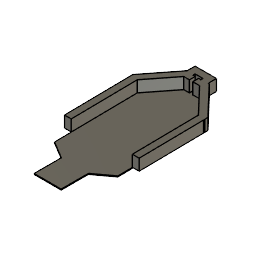
PCB CASE F3D (Autodesk Fusion 360 design; units mm, degrees)
part number: 2026-09-06-12-23-15-021
Autodesk Fusion 360 part; units mm, degrees
sketch "KiCad Dongle pcb-Edge_Cuts" plane through (0, 0, 0) normal (0, 0, 1) x (1, 0, 0)
  line L0 (141.0096, -48.4769) -> (141.0231, -48.4904)
  line L1 (141.0231, -48.4904) -> (141.025, -48.5)
  line L2 (141.025, -48.5) -> (141.025, -49.5)
  line L3 (141.025, -49.5) -> (141.0231, -49.5096)
  line L4 (141.0231, -49.5096) -> (141.0096, -49.5231)
  line L5 (141.0096, -49.5231) -> (141, -49.525)
  line L6 (141, -49.525) -> (140.025, -49.525)
  line L7 (140.025, -49.525) -> (140.025, -51.975)
  line L8 (140.025, -51.975) -> (143, -51.975)
  line L9 (143, -51.975) -> (143.0096, -51.9769)
  line L10 (143.0096, -51.9769) -> (143.0098, -51.9771)
  line L11 (143.0098, -51.9771) -> (143.0101, -51.9771)
  line L12 (143.0101, -51.9771) -> (143.0181, -51.9827)
  line L13 (143.0181, -51.9827) -> (154.0181, -63.4827)
  line L14 (154.0181, -63.4827) -> (154.0228, -63.4901)
  line L15 (154.0228, -63.4901) -> (154.0231, -63.4904)
  line L16 (154.0231, -63.4904) -> (154.0232, -63.4907)
  line L17 (154.0232, -63.4907) -> (154.0233, -63.4909)
  line L18 (154.0233, -63.4909) -> (154.0233, -63.4914)
  line L19 (154.0233, -63.4914) -> (154.025, -63.5)
  line L20 (154.025, -63.5) -> (154.025, -63.9998)
  line L21 (154.025, -63.9998) -> (154.4913, -99.4997)
  line L22 (154.4913, -99.4997) -> (154.4895, -99.5093)
  line L23 (154.4895, -99.5093) -> (154.488, -99.5108)
  line L24 (154.488, -99.5108) -> (154.4877, -99.5129)
  line L25 (154.4877, -99.5129) -> (154.4811, -99.5201)
  line L26 (154.4811, -99.5201) -> (147.025, -105.0126)
  line L27 (147.025, -105.0126) -> (147.025, -117)
  line L28 (147.025, -117) -> (147.0231, -117.0096)
  line L29 (147.0231, -117.0096) -> (147.0096, -117.0231)
  line L30 (147.0096, -117.0231) -> (147, -117.025)
  line L31 (147, -117.025) -> (135, -117.025)
  line L32 (135, -117.025) -> (134.9904, -117.0231)
  line L33 (134.9904, -117.0231) -> (134.9769, -117.0096)
  line L34 (134.9769, -117.0096) -> (134.975, -117)
  line L35 (134.975, -117) -> (134.975, -105.0142)
  line L36 (134.975, -105.0142) -> (127.4871, -100.5214)
  line L37 (127.4871, -100.5214) -> (127.4799, -100.5149)
  line L38 (127.4799, -100.5149) -> (127.4792, -100.512)
  line L39 (127.4792, -100.512) -> (127.477, -100.5099)
  line L40 (127.477, -100.5099) -> (127.475, -100.5003)
  line L41 (127.475, -100.5003) -> (126.975, -63.5003)
  line L42 (126.975, -63.5003) -> (126.9761, -63.4946)
  line L43 (126.9761, -63.4946) -> (126.9759, -63.4933)
  line L44 (126.9759, -63.4933) -> (126.9765, -63.4921)
  line L45 (126.9765, -63.4921) -> (126.9768, -63.4907)
  line L46 (126.9768, -63.4907) -> (126.9777, -63.4898)
  line L47 (126.9777, -63.4898) -> (126.9803, -63.4846)
  line L48 (126.9803, -63.4846) -> (135.9803, -51.9846)
  line L49 (135.9803, -51.9846) -> (135.9877, -51.9782)
  line L50 (135.9877, -51.9782) -> (135.9893, -51.978)
  line L51 (135.9893, -51.978) -> (135.9904, -51.9769)
  line L52 (135.9904, -51.9769) -> (136, -51.975)
  line L53 (136, -51.975) -> (138.475, -51.975)
  line L54 (138.475, -51.975) -> (138.475, -51.5)
  line L55 (138.475, -51.5) -> (138.475, -49.525)
  line L56 (138.475, -49.525) -> (137.5, -49.525)
  line L57 (137.5, -49.525) -> (137.4904, -49.5231)
  line L58 (137.4904, -49.5231) -> (137.4769, -49.5096)
  line L59 (137.4769, -49.5096) -> (137.475, -49.5)
  line L60 (137.475, -49.5) -> (137.475, -48.5)
  line L61 (137.475, -48.5) -> (137.4769, -48.4904)
  line L62 (137.4769, -48.4904) -> (137.4904, -48.4769)
  line L63 (137.4904, -48.4769) -> (137.5, -48.475)
  line L64 (137.5, -48.475) -> (141, -48.475)
  line L65 (141, -48.475) -> (141.0096, -48.4769)
  line L66 (137.525, -48.525) -> (137.525, -49.475)
  line L67 (137.525, -49.475) -> (138.5, -49.475)
  line L68 (138.5, -49.475) -> (138.5096, -49.4769)
  line L69 (138.5096, -49.4769) -> (138.5231, -49.4904)
  line L70 (138.5231, -49.4904) -> (138.525, -49.5)
  line L71 (138.525, -49.5) -> (138.525, -51.5)
  line L72 (138.525, -51.5) -> (138.525, -52)
  line L73 (138.525, -52) -> (138.5231, -52.0096)
  line L74 (138.5231, -52.0096) -> (138.5096, -52.0231)
  line L75 (138.5096, -52.0231) -> (138.5, -52.025)
  line L76 (138.5, -52.025) -> (136.0122, -52.025)
  line L77 (136.0122, -52.025) -> (127.0251, -63.5085)
  line L78 (127.0251, -63.5085) -> (127.5248, -100.4857)
  line L79 (127.5248, -100.4857) -> (135.0129, -104.9786)
  line L80 (135.0129, -104.9786) -> (135.0201, -104.9851)
  line L81 (135.0201, -104.9851) -> (135.0209, -104.9882)
  line L82 (135.0209, -104.9882) -> (135.0231, -104.9904)
  line L83 (135.0231, -104.9904) -> (135.025, -105)
  line L84 (135.025, -105) -> (135.025, -116.975)
  line L85 (135.025, -116.975) -> (146.975, -116.975)
  line L86 (146.975, -116.975) -> (146.975, -105)
  line L87 (146.975, -105) -> (146.9769, -104.9904)
  line L88 (146.9769, -104.9904) -> (146.9783, -104.989)
  line L89 (146.9783, -104.989) -> (146.9786, -104.9871)
  line L90 (146.9786, -104.9871) -> (146.9852, -104.9799)
  line L91 (146.9852, -104.9799) -> (154.4411, -99.4875)
  line L92 (154.4411, -99.4875) -> (153.975, -64.0003)
  line L93 (153.975, -64.0003) -> (153.975, -64.0002)
  line L94 (153.975, -64.0002) -> (153.975, -64)
  line L95 (153.975, -64) -> (153.975, -63.51)
  line L96 (153.975, -63.51) -> (142.9893, -52.025)
  line L97 (142.9893, -52.025) -> (140, -52.025)
  line L98 (140, -52.025) -> (139.9904, -52.0231)
  line L99 (139.9904, -52.0231) -> (139.9769, -52.0096)
  line L100 (139.9769, -52.0096) -> (139.975, -52)
  line L101 (139.975, -52) -> (139.975, -49.5)
  line L102 (139.975, -49.5) -> (139.9769, -49.4904)
  line L103 (139.9769, -49.4904) -> (139.9904, -49.4769)
  line L104 (139.9904, -49.4769) -> (140, -49.475)
  line L105 (140, -49.475) -> (140.975, -49.475)
  line L106 (140.975, -49.475) -> (140.975, -48.525)
  line L107 (140.975, -48.525) -> (137.525, -48.525)
extrude "Extrude1" add sketch "KiCad Dongle pcb-Edge_Cuts" along normal blind 0.4 contours L66 L67 L68 L69 L70 L71 L72 L73 L74 L75 L76 L77 L78 L79 L80 L81 L82 L83 L84 L85 L86 L87 L89 L90 L91 L92 L95 L96 L97 L98 L99 L100 L101 L102 L103 L104 L105 L106 L107 makes body 1
sketch "Sketch3" plane through (0, 0, 0.4) normal (0, 0, 1) x (-1, 0, 0)
  line L0 (-140.975, 48.525) -> (-137.525, 48.525)
  line L1 (-137.525, 48.525) -> (-137.525, 49.475)
  line L2 (-137.525, 49.475) -> (-138.5, 49.475)
  line L3 (-138.5, 49.475) -> (-138.5096, 49.4769)
  line L4 (-138.5096, 49.4769) -> (-138.5231, 49.4904)
  line L5 (-138.5231, 49.4904) -> (-138.525, 49.5)
  line L6 (-138.525, 49.5) -> (-138.525, 52)
  line L7 (-138.525, 52) -> (-138.5231, 52.0096)
  line L8 (-138.5231, 52.0096) -> (-138.5096, 52.0231)
  line L9 (-138.5096, 52.0231) -> (-138.5, 52.025)
  line L10 (-138.5, 52.025) -> (-136.0122, 52.025)
  line L11 (-136.0122, 52.025) -> (-127.0251, 63.5085)
  line L12 (-127.0251, 63.5085) -> (-127.5248, 100.4857)
  line L13 (-127.5248, 100.4857) -> (-135.0129, 104.9786)
  line L14 (-135.0129, 104.9786) -> (-135.0201, 104.9851)
  line L15 (-135.0201, 104.9851) -> (-135.0209, 104.9882)
  line L16 (-135.0209, 104.9882) -> (-135.0231, 104.9904)
  line L17 (-135.0231, 104.9904) -> (-135.025, 105)
  line L18 (-135.025, 105) -> (-135.025, 116.975)
  line L19 (-135.025, 116.975) -> (-146.975, 116.975)
  line L20 (-146.975, 116.975) -> (-146.975, 105)
  line L21 (-146.975, 105) -> (-146.9769, 104.9904)
  line L22 (-146.9769, 104.9904) -> (-146.9783, 104.989)
  line L23 (-146.9783, 104.989) -> (-146.9786, 104.9871)
  line L24 (-146.9786, 104.9871) -> (-146.9852, 104.9799)
  line L25 (-146.9852, 104.9799) -> (-154.4411, 99.4875)
  line L26 (-154.4411, 99.4875) -> (-153.975, 64.0003)
  line L27 (-153.975, 64.0003) -> (-153.975, 64.0002)
  line L28 (-153.975, 64.0002) -> (-153.975, 64)
  line L29 (-153.975, 64) -> (-153.975, 63.51)
  line L30 (-153.975, 63.51) -> (-142.9893, 52.025)
  line L31 (-142.9893, 52.025) -> (-140, 52.025)
  line L32 (-140, 52.025) -> (-139.9904, 52.0231)
  line L33 (-139.9904, 52.0231) -> (-139.9769, 52.0096)
  line L34 (-139.9769, 52.0096) -> (-139.975, 52)
  line L35 (-139.975, 52) -> (-139.975, 49.5)
  line L36 (-139.975, 49.5) -> (-139.9769, 49.4904)
  line L37 (-139.9769, 49.4904) -> (-139.9904, 49.4769)
  line L38 (-139.9904, 49.4769) -> (-140, 49.475)
  line L39 (-140, 49.475) -> (-140.975, 49.475)
  line L40 (-140.975, 49.475) -> (-140.975, 48.525)
  line L41 (-157.0281, 63.9788) -> (-156.975, 63.7083)
  line L42 (-156.975, 63.7083) -> (-156.975, 62.3063)
  line L43 (-156.975, 62.3063) -> (-144.2712, 49.025)
  line L44 (-144.2712, 49.025) -> (-143.975, 49.025)
  line L45 (-143.975, 49.025) -> (-143.975, 45.525)
  line L46 (-143.975, 45.525) -> (-134.525, 45.525)
  line L47 (-134.525, 45.525) -> (-134.525, 49.0576)
  line L48 (-134.525, 49.0576) -> (-124.0111, 62.492)
  line L49 (-124.0111, 62.492) -> (-124.5477, 102.198)
  line L50 (-124.5477, 102.198) -> (-132.025, 106.6844)
  line L51 (-132.025, 106.6844) -> (-132.025, 119.975)
  line L52 (-132.025, 119.975) -> (-149.975, 119.975)
  line L53 (-149.975, 119.975) -> (-149.975, 106.5035)
  line L54 (-149.975, 106.5035) -> (-157.4611, 100.9889)
  line L55 (-157.4611, 100.9889) -> (-156.9786, 64.2513)
  line L56 (-156.9786, 64.2513) -> (-157.0281, 63.9788)
  dimension "d8" = 3
extrude "Extrude2" add sketch "Sketch3" along normal blind 5 separate body makes body 2
split "Split1" by plane through (141, -116.975, 2.9) normal (0, -1, 0) bodies 2 makes body 3 at (138.0083, -119.975, 2.0667)
delete_body "RemoveBody1" bodies 3
box "BoxPrimitive2" cut length 13 width 7.601 height 7.601 placed x (0, -1, 0) y (1, 0, 0) z (0, 0, 1) at (127.3988, -106.6361, 0) bodies 2
box "BoxPrimitive3" cut length 10.426 width 10 height 1 placed x (0, 1, 0) y (-1, 0, 0) z (0, 0, 1) at (135, -117, 0) bodies 2
delete_face "DeleteFace1" 1 faces at (134.9998, -110.0824, 2.4667) on bodies 2
box "BoxPrimitive4" cut length 12.5 width 3.025 height -5.5 placed x (0, 1, 0) y (-1, 0, 0) z (0, 0, 1) at (150, -117.5, 5.4) bodies 2
box "BoxPrimitive5" cut length 1.51 width 11.814 height -5 placed x (0, 1, 0) y (-1, 0, 0) z (0, 0, 1) at (158.8136, -106.5103, 5.4) bodies 2
box "BoxPrimitive6" cut length 12 width 9 height -6 placed x (0, -1, 0) y (1, 0, 0) z (0, 0, 1) at (154.5185, -93.3748, 5.4) bodies 2
box "BoxPrimitive7" cut length 15 width 38 height 25 placed x (0, -1, 0) y (1, 0, 0) z (0, 0, 1) at (120, -93, 0) bodies 2
